Autodesk Inventor part; units mm, degrees
(part 2 of 2)
sketch "Sketch9" plane through (0, 2.54, 0) normal (0, 1, 0) x (1, 0, 0)
  line L0 (22.4402, 31.1118) -> (31.5374, 30.5468) projected
  line L1 (31.5374, 30.5468) -> (24.5097, 24.7424) projected
  line L2 (24.5097, 24.7424) -> (26.7836, 15.9159) projected
  line L3 (26.7836, 15.9159) -> (19.0916, 20.806) projected
  line L4 (19.0916, 20.806) -> (11.3997, 15.9159) projected
  line L5 (11.3997, 15.9159) -> (13.6736, 24.7424) projected
  line L6 (13.6736, 24.7424) -> (6.6459, 30.5468) projected
  line L7 (6.6459, 30.5468) -> (15.7431, 31.1118) projected
  line L8 (15.7431, 31.1118) -> (19.0916, 39.5891) projected
  line L9 (19.0916, 39.5891) -> (22.4402, 31.1118) projected
  line L10 (-16.7308, 13.6918) -> (-27.8255, 20.0974) projected
  line L11 (-27.8255, 20.0974) -> (-27.8255, 32.9084) projected
  line L12 (-27.8255, 32.9084) -> (-16.7308, 39.3139) projected
  line L13 (-16.7308, 39.3139) -> (-5.6361, 32.9084) projected
  line L14 (-5.6361, 32.9084) -> (-5.6361, 20.0974) projected
  line L15 (-5.6361, 20.0974) -> (-16.7308, 13.6918) projected
  circle A0 centre (0, 0) radius 50.8 projected
  line L16 (22.0447, 4.397) -> (22.0447, 5.9805) projected
  line L17 (22.0447, 5.9805) -> (31.5841, 5.9805) projected
  line L18 (31.5841, 5.9805) -> (32.8893, 2.3625) projected
  line L19 (32.8893, 2.3625) -> (31.4017, 1.825) projected
  line L20 (27.9852, 4.1475) -> (26.2386, 4.1475) projected
  line L21 (26.2386, 4.1475) -> (26.2386, 1.2972) projected
  line L22 (26.2386, 1.2972) -> (26.8144, 1.2972) projected
  line L23 (28.11, 2.4872) -> (28.11, 2.9191) projected
  line L24 (28.11, 2.9191) -> (29.5687, 2.9191) projected
  line L25 (29.5687, 2.9191) -> (29.5687, -1.9178) projected
  line L26 (29.5687, -1.9178) -> (28.11, -1.9178) projected
  line L27 (28.11, -1.9178) -> (28.11, -1.4283) projected
  line L28 (26.7568, -0.2959) -> (26.2386, -0.2959) projected
  line L29 (26.2386, -0.2959) -> (26.2386, -2.9159) projected
  line L30 (26.9487, -3.6164) -> (27.9084, -3.6164) projected
  line L31 (31.9296, -0.6894) -> (33.4267, -1.198) projected
  line L32 (33.4267, -1.198) -> (31.9296, -5.4495) projected
  line L33 (31.9296, -5.4495) -> (22.0447, -5.4495) projected
  line L34 (22.0447, -5.4495) -> (22.0447, -3.866) projected
  line L35 (22.0447, -3.866) -> (22.3326, -3.866) projected
  line L36 (23.4171, -2.8007) -> (23.4171, 3.4181) projected
  line L37 (22.5533, 4.397) -> (22.0447, 4.397) projected
  line L38 (-2.1013, 4.397) -> (-2.1013, 5.9805) projected
  line L39 (-2.1013, 5.9805) -> (2.5244, 5.9805) projected
  line L40 (2.5244, 5.9805) -> (5.8834, -0.6894) projected
  line L41 (5.8834, -0.6894) -> (5.8834, 3.3893) projected
  line L42 (5.0676, 4.397) -> (4.511, 4.397) projected
  line L43 (4.511, 4.397) -> (4.511, 5.9805) projected
  line L44 (4.511, 5.9805) -> (9.2135, 5.9805) projected
  line L45 (9.2135, 5.9805) -> (9.2135, 4.397) projected
  line L46 (9.2135, 4.397) -> (8.6953, 4.397) projected
  line L47 (7.8412, 3.3893) -> (7.8412, -5.4495) projected
  line L48 (7.8412, -5.4495) -> (5.4899, -5.4495) projected
  line L49 (5.4899, -5.4495) -> (1.248, 2.9767) projected
  line L50 (1.248, 2.9767) -> (1.248, -2.9159) projected
  line L51 (2.0734, -3.866) -> (2.6204, -3.866) projected
  line L52 (2.6204, -3.866) -> (2.6204, -5.4495) projected
  line L53 (2.6204, -5.4495) -> (-2.1013, -5.4495) projected
  line L54 (-2.1013, -5.4495) -> (-2.1013, -3.866) projected
  line L55 (-2.1013, -3.866) -> (-1.6119, -3.866) projected
  line L56 (-0.7289, -3.0406) -> (-0.7289, 3.5141) projected
  line L57 (-1.4967, 4.397) -> (-2.1013, 4.397) projected
  line L58 (-45.4605, 4.397) -> (-45.4605, 5.9805) projected
  line L59 (-45.4605, 5.9805) -> (-39.8942, 5.9805) projected
  line L60 (-39.8942, 5.9805) -> (-39.8942, 4.397) projected
  line L61 (-39.8942, 4.397) -> (-40.4028, 4.397) projected
  line L62 (-41.2666, 3.4277) -> (-41.2666, -2.8871) projected
  line L63 (-40.4988, -3.866) -> (-39.8942, -3.866) projected
  line L64 (-39.8942, -3.866) -> (-39.8942, -5.4495) projected
  line L65 (-39.8942, -5.4495) -> (-45.4605, -5.4495) projected
  line L66 (-45.4605, -5.4495) -> (-45.4605, -3.866) projected
  line L67 (-45.4605, -3.866) -> (-45.0094, -3.866) projected
  line L68 (-44.0881, -2.9734) -> (-44.0881, 3.3702) projected
  line L69 (-44.9518, 4.397) -> (-45.4605, 4.397) projected
  line L70 (-32.946, 4.397) -> (-32.946, 5.9805) projected
  line L71 (-32.946, 5.9805) -> (-26.9095, 5.9805) projected
  line L72 (-26.8039, -0.9197) -> (-28.7521, -0.9197) projected
  line L73 (-28.7521, -0.9197) -> (-28.7521, -3.0598) projected
  line L74 (-27.9556, -3.866) -> (-27.3797, -3.866) projected
  line L75 (-27.3797, -3.866) -> (-27.3797, -5.4495) projected
  line L76 (-27.3797, -5.4495) -> (-32.946, -5.4495) projected
  line L77 (-32.946, -5.4495) -> (-32.946, -3.866) projected
  line L78 (-32.946, -3.866) -> (-32.5621, -3.866) projected
  line L79 (-31.5736, -2.8967) -> (-31.5736, 3.3798) projected
  line L80 (-32.399, 4.397) -> (-32.946, 4.397) projected
  line L81 (-21.9383, 4.349) -> (-21.9383, 5.9805) projected
  line L82 (-21.9383, 5.9805) -> (-14.8941, 5.9805) projected
  line L83 (-13.7041, -0.3439) -> (-11.3528, -3.079) projected
  line L84 (-11.3528, -3.079) -> (-11.2568, -3.2038) projected
  line L85 (-9.9324, -3.866) -> (-9.443, -3.866) projected
  line L86 (-9.443, -3.866) -> (-9.443, -5.4495) projected
  line L87 (-9.443, -5.4495) -> (-13.109, -5.4495) projected
  line L88 (-13.109, -5.4495) -> (-16.7751, -0.5262) projected
  line L89 (-16.7751, -0.5262) -> (-17.7252, -0.5262) projected
  line L90 (-17.7252, -0.5262) -> (-17.7252, -2.8007) projected
  line L91 (-16.8711, -3.866) -> (-16.3528, -3.866) projected
  line L92 (-16.3528, -3.866) -> (-16.3528, -5.4495) projected
  line L93 (-16.3528, -5.4495) -> (-21.9383, -5.4495) projected
  line L94 (-21.9383, -5.4495) -> (-21.9383, -3.866) projected
  line L95 (-21.9383, -3.866) -> (-21.4296, -3.866) projected
  line L96 (-20.5659, -2.9063) -> (-20.5659, 3.5237) projected
  line L97 (-21.2761, 4.3586) -> (-21.5064, 4.349) projected
  line L98 (-21.5064, 4.349) -> (-21.9383, 4.349) projected
  line L99 (-8.896, 4.397) -> (-8.896, 5.9805) projected
  line L100 (-8.896, 5.9805) -> (-3.3297, 5.9805) projected
  line L101 (-3.3297, 5.9805) -> (-3.3297, 4.397) projected
  line L102 (-3.3297, 4.397) -> (-3.8384, 4.397) projected
  line L103 (-4.7021, 3.4277) -> (-4.7021, -2.8871) projected
  line L104 (-3.9343, -3.866) -> (-3.3297, -3.866) projected
  line L105 (-3.3297, -3.866) -> (-3.3297, -5.4495) projected
  line L106 (-3.3297, -5.4495) -> (-8.896, -5.4495) projected
  line L107 (-8.896, -5.4495) -> (-8.896, -3.866) projected
  line L108 (-8.896, -3.866) -> (-8.4449, -3.866) projected
  line L109 (-7.5236, -2.9734) -> (-7.5236, 3.3702) projected
  line L110 (-8.3873, 4.397) -> (-8.896, 4.397) projected
  line L111 (9.6742, 2.3529) -> (11.0849, 6.3644) projected
  line L112 (11.0849, 6.3644) -> (12.1598, 6.3644) projected
  line L113 (12.1598, 6.3644) -> (12.275, 5.9805) projected
  line L114 (12.275, 5.9805) -> (18.7241, 5.9805) projected
  line L115 (18.7241, 5.9805) -> (18.8585, 6.3644) projected
  line L116 (18.8585, 6.3644) -> (19.9429, 6.3644) projected
  line L117 (19.9429, 6.3644) -> (21.3633, 2.3529) projected
  line L118 (21.3633, 2.3529) -> (19.8374, 1.825) projected
  line L119 (16.9199, 3.802) -> (16.9199, -2.7623) projected
  line L120 (18.2923, -3.866) -> (18.2923, -5.4495) projected
  line L121 (18.2923, -5.4495) -> (12.726, -5.4495) projected
  line L122 (12.726, -5.4495) -> (12.726, -3.866) projected
  line L123 (12.726, -3.866) -> (13.0619, -3.866) projected
  line L124 (14.0984, -2.8199) -> (14.0984, 3.898) projected
  line L125 (11.1713, 1.825) -> (9.6742, 2.3529) projected
  line L126 (34.0985, 4.397) -> (34.0985, 5.9805) projected
  line L127 (34.0985, 5.9805) -> (40.087, 5.9805) projected
  line L128 (39.3768, -5.4495) -> (34.0985, -5.4495) projected
  line L129 (34.0985, -5.4495) -> (34.0985, -3.866) projected
  line L130 (34.0985, -3.866) -> (34.492, -3.866) projected
  line L131 (35.4709, -2.8295) -> (35.4709, 3.4181) projected
  line L132 (34.492, 4.397) -> (34.0985, 4.397) projected
  constraints: 55 other
extrude "Extrusion8" add sketch "Sketch9" against normal blind 2.54 separate body contours L0 L1 L2 L3 L4 L5 L6 L7 L8 L9
body "Solid1"
body "Solid2"
body "Solid3"
body "Solid4"
body "Solid5"
body "Solid6"
